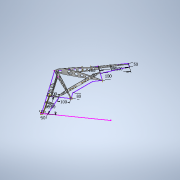
# Autodesk Inventor part: aile1
Saved by Autodesk Inventor 2020 (Build 240168000, 168)
## iProperties
Created: 2019-12-13
Part Number: aile1
Material: Générique
Document SubType Name: Modeling
Designer: guill
Density: 1 g/cm^3
Appearance: Par défaut
Author: guill
Autodesk Inventor part; units mm, degrees
ref_plane "YZ Plane" through (0, 0, 0) normal (1, 0, 0) x (0, 1, 0)
sketch "Esquisse1" plane through (0, 0, 0) normal (0, 1, 0) x (-1, 0, 0)
  line L0 (0, 0) -> (-350.103769, 500)
  line L1 (0, 0) -> (-350.103769, -500)
  line L2 (-350.103769, 500) -> (-178.030838, 254.254387)
  line L3 (-350.103769, -500) -> (-178.030838, -254.254387)
  line L4 (-350.103769, 500) -> (-391.061371, 471.321178)
  line L5 (-350.103769, -500) -> (-391.061371, -471.321178)
  line L6 (-350.103769, 500) -> (-206.70966, 295.211989)
  line L7 (-206.70966, 295.211989) -> (-288.624864, 237.854345)
  line L8 (-288.624864, 237.854345) -> (-391.061371, 471.321178)
  line L9 (-350.103769, -500) -> (-206.70966, -295.211989)
  line L10 (-206.70966, -295.211989) -> (-288.624864, -237.854345)
  line L11 (-288.624864, -237.854345) -> (-391.061371, -471.321178)
  line L12 (-288.624864, 237.854345) -> (-370.540069, 180.496702)
  line L13 (-288.624864, -237.854345) -> (-370.540069, -180.496702)
  line L14 (-370.540069, -180.496702) -> (-324.653954, -114.964538)
  line L15 (-370.540069, 180.496702) -> (-324.653954, 114.964538)
  line L16 (-370.540069, 180.496702) -> (-324.653954, 114.964538)
  line L17 (-324.653954, 114.964538) -> (-324.653954, -114.964538)
  dimension "d19" = 50
  dimension "d20" = 90
  dimension "d21" = 50
  dimension "d22" = 90
  dimension "d23" = 250
  dimension "d24" = 100
  dimension "d25" = 250
  dimension "d26" = 100
  dimension "d27" = 100
  dimension "d28" = 100
  dimension "d29" = 80
  constraints: 36 end point, 4 point on line, 3 perpendicular, 1 vertical
  measures "d19" distance of L0.end L4.end
  measures "d20" angle of L0 L4
  measures "d21" distance of L1.end L5.end
  measures "d22" angle of L1 L5
  measures "d23" distance of L0.end L6.end
  measures "d24" distance of L6.end L7.end
  measures "d25" distance of L1.end L9.end
  measures "d26" distance of L9.end L10.end
  measures "d27" distance of L7.end L12.end
  measures "d28" distance of L10.end L13.end
  measures "d29" distance of L15.end L12.end
ref_plane "Plan de construction11" through (370.540069, 0, 180.496702) normal (0.5735764, 0, 0.819152) x (0.819152, 0, -0.5735764)
sketch "Esquisse3" plane through (370.540069, 0, 180.496702) normal (0.5735764, 0, 0.819152) x (0.819152, 0, -0.5735764)
  line L0 (0, 1) -> (-100, 1)
  line L1 (-200, 0) -> (-200, 1)
  line L2 (-200, 1) -> (-175, 1)
  line L3 (373.576436, 1) -> (-200, 1)
  line L4 (-175, 1) -> (-175, 16)
  line L5 (-175, 16) -> (-193.067438, 16)
  line L6 (-193.067438, 16) -> (-175, 16)
  arc A0 (-175, 16) -> (-200, 1) centre (-175, -12.333333) ccw
  arc A1 (-100, 1) -> (-175, 16) centre (-175, -179) ccw
  line L7 (-175, 1) -> (-175, -4)
  line L8 (-175, -4) -> (-209.42791, -4)
  line L9 (-209.42791, -4) -> (-116.779842, -4)
  arc A2 (-200, 1) -> (-175, -4) centre (-175, 61) ccw
  arc A3 (-175, -4) -> (-100, 1) centre (-175, 561) ccw
  line L10 (-200, 1) -> (-175, 8.5)
  line L11 (-100, 0) -> (-100, 1)
  line L12 (-175, 8.5) -> (-100, 1)
  circle A4 centre (-187, 4.9) radius 5
  circle A5 centre (-163, 7.3) radius 6.5
  circle A6 centre (-148.074442, 5.807444) radius 5.5
  circle A7 centre (-133.074442, 4.307444) radius 4.5
  circle A8 centre (-121.074442, 3.107444) radius 3
  line L13 (-175, 16) -> (-175, 8.5)
  line L14 (-178, 9.840729) -> (-178, 15.840729)
  line L15 (-178, 9.840729) -> (-175, 9.840729)
  line L16 (-175, 16) -> (-175, 9.840729)
  line L17 (-178, 9.840729) -> (-178, -3.895538)
  line L18 (-178, -3.895538) -> (-178, 9.840729)
  line L19 (-175, 9.840729) -> (-175, -4)
  line L20 (-105.241635, 0.322936) -> (-103.229356, 0.322936)
  line L21 (-103.229356, 0.322936) -> (-105.241635, 0.322936)
  line L22 (-105.241635, 0.322936) -> (-105.135598, 0.322936)
  line L23 (-178, 1) -> (-178, -3.895538)
  line L24 (-175, 1) -> (-175, -4)
  line L25 (-178, 1) -> (-178, -3.895538)
  line L26 (-178, -3.603939) -> (-178, 1)
  point P0 (-178, 1)
  point P1 (-175, 9.840729)
  dimension "d36" = 100
  dimension "d37" = 25
  dimension "d38" = 15
  dimension "d40" = 5
  dimension "d94" = 13
  dimension "d95" = 11
  dimension "d96" = 9
  dimension "d97" = 10
  dimension "d98" = 12
  dimension "d99" = 12
  dimension "d100" = 15
  dimension "d101" = 15
  dimension "d102" = 6
  dimension "d103" = 12
  dimension "d104" = 6
  dimension "d105" = 3
  constraints: 48 end point, 14 point on line, 12 point on circle, 9 centre point, 7 collinear, 4 horizontal, 4 tangent, 3 perpendicular, 2 vertical, 1 midpoint, 1 parallel
  measures "d36" distance of L0.start L0.end
  measures "d37" distance of L1.end L2.end
  measures "d38" distance of L2.end L4.end
  measures "d40" distance of L2.end L7.end
  measures "d94" diameter of A5
  measures "d95" diameter of A6
  measures "d96" diameter of A7
  measures "d97" diameter of A4
  measures "d98" distance from line of L4 A4.centre
  measures "d99" distance from line of A5.centre L4
  measures "d100" distance of A5.centre A6.centre
  measures "d101" horizontal distance of A7.centre A6.centre
  measures "d102" diameter of A8
  measures "d103" horizontal distance of A8.centre A7.centre
  measures "d104" distance of L14.start L14.end
  measures "d105" distance of L14.start L15.end
ref_plane "Plan de construction9" through (370.540069, 0, -180.496702) normal (0.5735764, 0, -0.819152) x (-0.819152, 0, -0.5735764)
sketch "Esquisse6" plane through (370.540069, 0, -180.496702) normal (0.5735764, 0, -0.819152) x (-0.819152, 0, -0.5735764)
  point P0 (200, 0)
ref_plane "Plan de construction10" through (0, 1, 0) normal (0, 1, 0) x (1, 0, 0)
sketch "Esquisse7" plane through (0, 1, 0) normal (0, 1, 0) x (1, 0, 0)
  point P0 (0, 0)
ref_plane "Plan de construction12" through (350.103769, 0, 500) normal (0.5735764, 0, 0.819152) x (0.819152, 0, -0.5735764)
sketch "Esquisse9" plane through (350.103769, 0, 500) normal (0.5735764, 0, 0.819152) x (0.819152, 0, -0.5735764)
  line L0 (0.030028, 1) -> (15.030028, 1)
  line L1 (573.576436, 1) -> (0, 1)
  line L2 (0, 0) -> (50, 0)
  line L3 (0, 0) -> (15.030028, 0)
  line L4 (0, 1) -> (50, 1)
  line L5 (15.030028, 0) -> (15.030028, 1)
  dimension "d44" = 15
  constraints: 6 end point, 1 parallel, 1 perpendicular, 1 point on line
  measures "d44" distance of L0.start L0.end
ref_plane "Plan de construction4" through (228.90919, 16, 283.330034) normal (-0.8416187, 0, 0.5400722) x (0, -1, 0)
sketch "Esquisse10" plane through (228.90919, 16, 283.330034) normal (-0.8416187, 0, 0.5400722) x (0, -1, 0)
  ellipse E0 centre (-545, 0) end of major axis (20, 0) minor radius 22.787252 (16, -2.706716) -> (20, 0) ccw
  line L0 (-0.227332, -2.706716) -> (16, -2.706716)
  line L1 (0, -2.997559) -> (0, 0)
  line L2 (0, 0) -> (20, 0)
  line L3 (14.969754, 247.211181) -> (16, 247.211181)
  arc A0 (14.969754, 247.211181) -> (0, 0) centre (1799.771575, 15.074532) ccw
  arc A1 (20, 0) -> (16, 247.211181) centre (-6662.887369, 15.505506) ccw
  line L4 (10, 0) -> (14.969754, 247.211181)
  circle A2 centre (10.265058, 13.184834) radius 6.5
  circle A3 centre (10.667124, 33.184834) radius 6.5
  circle A4 centre (11.049086, 52.184834) radius 6
  circle A5 centre (11.390842, 69.184834) radius 5.5
  circle A6 centre (11.712494, 85.184834) radius 5
  circle A7 centre (12.11456, 105.184834) radius 5
  circle A8 centre (12.436212, 121.184834) radius 4.5
  circle A9 centre (12.737761, 136.184834) radius 4
  circle A10 centre (13.03931, 151.184834) radius 3.5
  circle A11 centre (13.320756, 165.184834) radius 3.5
  circle A12 centre (13.582099, 178.184834) radius 3
  circle A13 centre (14.044474, 201.184834) radius 1.5
  circle A14 centre (13.823338, 190.184834) radius 2.5
  line L5 (1.668204, 94) -> (7.951039, 94)
  line L6 (15, 245.790745) -> (15, -6.022415)
  line L7 (7.951039, 94) -> (7.951039, 97)
  line L8 (7.951039, 97) -> (1.802392, 97)
  ellipse E1 centre (28.333333, 0) end of major axis (0, 0) minor radius 1.142724 (15, 1.008285) -> (0, 0) ccw
  line L9 (15, 1.008285) -> (0, -2.997559)
  line L10 (0, -2.997559) -> (6, -2.997559)
  line L11 (6, -2.997559) -> (6, 0)
  line L12 (0, 0) -> (0, -2.997559)
  ellipse E2 centre (195, 0) end of major axis (0, 0) minor radius 7.864627 (0, 0) -> (15, -3.024856) ccw
  line L13 (0, 0) -> (6, 0)
  line L14 (16, 245.790745) -> (16, -6.022415)
  line L15 (6, 0) -> (6, -2.997559)
  line L16 (15, -3.000658) -> (15, 1.008285)
  line L17 (6, -2.997559) -> (6, 0)
  ellipse E3 centre (28.333333, -2.997559) end of major axis (0, -2.997559) minor radius 1.142724 (15, -1.989274) -> (0, -2.997559) ccw
  line L18 (0, 0) -> (6, 0)
  ellipse E4 centre (195, -2.997559) end of major axis (0, -2.997559) minor radius 7.864627 (0, -2.997559) -> (15, -6.022415) ccw
  line L19 (10, 0) -> (6, 0)
  point P0 (16, -362.083342)
  point P1 (10.134413, 6.686147)
  point P2 (10.395703, 19.683521)
  point P3 (10.536479, 26.686147)
  point P4 (10.797769, 39.683521)
  point P5 (10.928491, 46.186046)
  point P6 (11.169681, 58.183622)
  point P7 (11.280296, 63.685945)
  point P8 (11.501387, 74.683723)
  point P9 (11.611998, 80.185844)
  point P10 (11.81299, 90.183824)
  point P11 (12.014063, 100.185844)
  point P12 (12.215056, 110.183824)
  point P13 (12.345765, 116.685743)
  point P14 (12.526658, 125.683925)
  point P15 (12.657364, 132.185642)
  point P16 (12.818158, 140.184026)
  point P17 (12.968963, 147.685541)
  point P18 (13.109657, 154.684127)
  point P19 (13.250409, 161.685541)
  point P20 (13.391103, 168.684127)
  point P21 (13.521801, 175.18544)
  point P22 (13.642396, 181.184228)
  point P23 (13.77309, 187.685339)
  point P24 (13.873586, 192.684329)
  point P25 (14.014325, 199.685137)
  point P26 (15, 200.02856)
  point P27 (15, 192.390614)
  point P28 (15, 187.979054)
  point P29 (15, 180.828611)
  point P30 (15, 175.541057)
  point P31 (15, 168.255687)
  point P32 (15, 162.113981)
  point P33 (15, 154.084092)
  point P34 (15, 148.285576)
  point P35 (15, 139.483663)
  point P36 (15, 132.886005)
  point P37 (15, 124.883076)
  point P38 (15, 117.486592)
  point P39 (15, 109.268243)
  point P40 (15, 101.101424)
  point P41 (15, 88.952101)
  point P42 (15, 81.417566)
  point P43 (15, 73.335012)
  point P44 (15, 65.034656)
  point P45 (15, 56.700394)
  point P46 (15, 47.669274)
  point P47 (15, 38.030057)
  point P48 (15, 28.339611)
  point P49 (15, 17.63796)
  point P50 (15, 8.731708)
  point P51 (15, 0)
  dimension "d51" = 13
  dimension "d52" = 13
  dimension "d53" = 12
  dimension "d54" = 13.18483
  dimension "d55" = 11
  dimension "d56" = 10
  dimension "d57" = 10
  dimension "d58" = 9
  dimension "d59" = 8
  dimension "d60" = 7
  dimension "d61" = 3
  dimension "d62" = 5
  dimension "d63" = 6
  dimension "d64" = 7
  dimension "d65" = 14
  dimension "d66" = 13
  dimension "d67" = 12
  dimension "d68" = 11
  dimension "d69" = 15
  dimension "d70" = 15
  dimension "d71" = 16
  dimension "d72" = 20
  dimension "d73" = 16
  dimension "d74" = 17
  dimension "d75" = 19
  dimension "d76" = 20
  dimension "d77" = 247.21118
  dimension "d78" = 3
  dimension "d79" = 94
  dimension "d106" = 6
  constraints: 30 end point, 15 centre point, 6 point on circle, 5 horizontal, 4 perpendicular, 3 vertical, 2 collinear, 1 midpoint, 1 parallel, 1 point on line, 22 other
  measures "d51" diameter of A2
  measures "d52" diameter of A3
  measures "d53" diameter of A4
  measures "d54" vertical distance of A2.centre L19.start
  measures "d55" diameter of A5
  measures "d56" diameter of A6
  measures "d57" diameter of A7
  measures "d58" diameter of A8
  measures "d59" diameter of A9
  measures "d60" diameter of A10
  measures "d61" diameter of A13
  measures "d62" diameter of A14
  measures "d63" diameter of A12
  measures "d64" diameter of A11
  measures "d65" vertical distance of A11.centre A10.centre
  measures "d66" vertical distance of A12.centre A11.centre
  measures "d67" vertical distance of A14.centre A12.centre
  measures "d68" vertical distance of A14.centre A13.centre
  measures "d69" vertical distance of A10.centre A9.centre
  measures "d70" vertical distance of A9.centre A8.centre
  measures "d71" vertical distance of A8.centre A7.centre
  measures "d72" vertical distance of A7.centre A6.centre
  measures "d73" vertical distance of A5.centre A6.centre
  measures "d74" vertical distance of A5.centre A4.centre
  measures "d75" vertical distance of A3.centre A4.centre
  measures "d76" vertical distance of A3.centre A2.centre
  measures "d77" distance between parallel lines of L2 L3
  measures "d78" distance from line of L8 L5.start
  measures "d79" distance between parallel lines of L2 L5
  measures "d106" distance of L1.start L10.end
extrude "Extrusion4" add sketch "Esquisse10" along normal blind 3 contours L2 L14 A2 A3 A4 A5 A6 A7 A8 A9 A10 A11 A12 A14 L6 A13 L4 L3 A1 | L2 L6 A2 L14 | L2 L9 L6 | L4 A13 A14 A12 A11 A10 A9 A8 A7 A6 A5 A4 A3 A2 E1 A0 L5 L7 L8 | L11 L10 L9 L0 | L0 L9 E3 L11 | L2 L4 E1 L9 | E1 L4 A2 L6 | A2 L6 A3 L14 | L9 E3 L0 | L0 E3 L9 | E3 L9 E2 L11 | E2 L9 L11 | L2 E1 L4 | L9 E2 L2 L11 | A2 L4 A3 L6 | A13 L6 A14 L4 | E3 L1 L0 | L0 L1 E2 L9 E3 | A3 L6 A4 L14 | A3 L4 A4 L6 | A14 L6 A12 L4 | A4 L6 A5 L14 | A14 L14 A12 L6 | A4 L4 A5 L6 | A12 L6 A11 L4 | A5 L6 A6 L14 | A12 L14 A11 L6 | A5 L4 A6 L6 | A11 L6 A10 L4 | A6 L6 A7 L14 | A11 L14 A10 L6 | A6 L4 A7 L6 | A10 L6 A9 L4 | A7 L6 A8 L14 | A10 L14 A9 L6 | A7 L4 A8 L6 | A9 L6 A8 L4 | A8 L6 A9 L14
sketch "Esquisse11" plane through (279.675976, 8.048961, 362.442192) normal (0.5400722, 0, 0.8416187) x (0.8416187, 0, -0.5400722)
  line L0 (-3, -8.761455) -> (-3, 7.791507)
  line L1 (-3, 6.274364) -> (-3, 6.175837)
  line L2 (66.936248, -8.048961) -> (-22.552672, -8.048961)
  line L3 (-3, 0.174364) -> (-0.027124, 0.174364)
  line L4 (-0.027124, 6.274364) -> (-3, 6.274364)
  line L5 (0, -8.81402) -> (0, 4.18598)
  line L6 (-20.949217, 6.274364) -> (-3, 6.274364)
  line L7 (-39.635584, -7.048961) -> (-15.017799, -7.048961)
  arc A0 (-0.027124, 6.274364) -> (-21.3, -7.048961) centre (-1.513562, -14.996777) ccw
  line L8 (-25.100653, -7.048961) -> (74.817983, -7.048961)
  arc A1 (58.967528, -7.048961) -> (-0.027124, 6.274364) centre (2.642517, -119.178211) ccw
  line L9 (-39.635584, -8.048961) -> (-15.017799, -8.048961)
  line L10 (0, -8.048961) -> (0, -12.066949)
  line L11 (-21.3, -7.048961) -> (-21.3, -8.048961)
  line L12 (-3, -11.509391) -> (0, -11.509391)
  line L13 (6.100773, -11.509391) -> (0, -11.509391)
  arc A2 (-21.3, -8.048961) -> (0, -11.509391) centre (-1.5, 46.541859) ccw
  arc A3 (0, -11.509391) -> (58.967528, -8.048961) centre (2.772798, 445.389574) ccw
  line L14 (58.967528, -7.048961) -> (58.967528, -8.048961)
  ellipse E0 centre (-0.120994, -187.048961) end of major axis (-0.120994, 7.951039) minor radius 194.84134 (74.817983, -7.048961) -> (-0.120994, 7.951039) ccw
  line L15 (0, -1.842696) -> (58.967528, -7.048961)
  circle A4 centre (9, -2.63731) radius 5.5
  circle A5 centre (24, -3.961665) radius 4.5
  circle A6 centre (39, -5.286021) radius 3.5
  line L16 (-21.3, -7.048961) -> (-3, -1.811706)
  line L17 (-3, -8.761455) -> (-3, 1.238545)
  circle A7 centre (-11, -4.101217) radius 4.5
  line L18 (-3, -11.509391) -> (-3, 0.174364)
  line L19 (-0.027124, 0.174364) -> (0, -11.509391)
  line L20 (56.859742, -6.862864) -> (56.859742, -8.048961)
  line L21 (58.967528, -8.048961) -> (56.859742, -8.048961)
  line L22 (56.859742, -6.862864) -> (56.859742, -8.048961)
  point P0 (-24.979659, -7.048961)
  point P1 (-25.100653, -7.048961)
  point P2 (0, -12.048961)
  point P3 (-3, -8.761455)
  point P4 (-3, 0.174364)
  point P5 (-0.008033, -8.048961)
  point P6 (5.545597, -11.509391)
  dimension "d82" = 6.1
  dimension "d83" = 18.3
  dimension "d84" = 11
  dimension "d85" = 9
  dimension "d86" = 7
  dimension "d87" = 15
  dimension "d88" = 15
  dimension "d89" = 9
  dimension "d90" = 8
  dimension "d91" = 9
  constraints: 30 end point, 14 point on line, 11 point on circle, 8 centre point, 5 perpendicular, 4 vertical, 2 collinear, 1 horizontal, 6 other
  measures "d82" distance of L1.start L3.start
  measures "d83" distance between parallel lines of L0 L11
  measures "d84" diameter of A4
  measures "d85" diameter of A5
  measures "d86" diameter of A6
  measures "d87" horizontal distance of A5.centre A4.centre
  measures "d88" horizontal distance of A6.centre A5.centre
  measures "d89" diameter of A7
  measures "d90" distance from line of A7.centre L17
extrude "Extrusion5" add sketch "Esquisse11" along normal blind 3 contours L16 A7 A0 L0 | L0 L8 A7 L16 | L0 L4 A1 L15 A6 A5 A4 L5 L8 L19 L3 | L0 L2 A7 L8 | L0 L18 A2 L2 A7 | L8 L5 L2 L19 | A7 L8 L7 L16 | A7 L2 L11 L7 L8 | L8 A4 L2 L5 | L5 L15 A4 L8 | L2 A4 A5 A6 A3 L13 L10 L5 | A4 L15 A5 L8 | L8 A5 L2 A4 | L20 L2 A6 L8 | L8 A6 L15 L20 | A5 L15 A6 L8 | L8 A6 L2 A5
extrude "Extrusion6" add sketch "Esquisse3" along normal blind 3 contours L17 L10 L4 L2 | L2 L7 A2 A4 | L2 A4 L10 L17 | L4 L12 A5 L3 | L3 A5 A6 A7 A8 A3 L7 | L17 L15 L4 L10 | L10 A4 A0 L14 L17 | L4 A1 L12 A8 A7 A6 A5 | L2 L10 A4 | A5 L12 A6 L3 | L3 A8 L12 | A6 L12 A7 L3 | L3 A7 L12 A8 picked at (-194.398279, 2.332998) picked at (-112.107283, 1.985135)
ref_plane "Plan de construction5" through (0, 1, 0) normal (0.4379247, 0, -0.8990117) x (0.8990117, 0, 0.4379247)
sketch "Esquisse12" plane through (0, 1, 0) normal (0.4379247, 0, -0.8990117) x (0.8990117, 0, 0.4379247)
  line L0 (0, 0) -> (315.115011, 0)
  line L1 (0, 0) -> (90, 0)
  line L2 (90, 0) -> (90, -40)
  line L3 (0, 1) -> (0, 0)
  line L4 (0, 0) -> (90, 0)
  line L5 (90, 1) -> (90, 16)
  line L6 (90, -40) -> (64.056463, -40)
  arc A0 (0, 0) -> (90, -40) centre (90, 81.25) ccw
  line L7 (90, 16) -> (68.484817, 16)
  arc A1 (90, 16) -> (0, 1) centre (86.556789, -240.840731) ccw
  line L8 (90, -40) -> (109.634057, -40)
  line L9 (363.639408, 1) -> (412.163805, 1)
  arc A2 (90, -40) -> (412.163805, 1) centre (99.817028, 1169.087008) ccw
  line L10 (90, 16) -> (104.02297, 16)
  line L11 (0, 0) -> (90, -17.116159)
  line L12 (90, -17.116159) -> (384.32761, 1)
  line L13 (412.163805, 1) -> (342.2135, 1)
  circle A3 centre (50, -9.508977) radius 16.5
  circle A4 centre (135, -14.346364) radius 20
  circle A5 centre (190, -10.961059) radius 15
  circle A6 centre (237.163805, -8.05808) radius 13.5
  circle A7 centre (282.163805, -5.288285) radius 12.5
  circle A8 centre (322.163805, -2.826244) radius 8.5
  line L14 (412.163805, 1) -> (412.163805, 0)
  line L15 (90, 0) -> (90, 21.872289)
  line L16 (0, 1) -> (399.114343, 1)
  line L17 (90, 16) -> (105.35625, 16)
  line L18 (105.35625, 16) -> (90, 16)
  arc A9 (412.163805, 1) -> (90, 16) centre (97.011485, -3300.56079) ccw
  line L19 (314.469379, -20.834055) -> (314.469379, -10.834055)
  line L20 (314.469379, -10.834055) -> (311.469379, -10.834055)
  line L21 (311.469379, -10.834055) -> (311.469379, -21.371328)
  point P0 (104.02297, 16)
  point P1 (83.113577, 16)
  dimension "d110" = 90
  dimension "d111" = 315.11501
  dimension "d112" = 40
  dimension "d113" = 90
  dimension "d114" = 90
  dimension "d115" = 15
  dimension "d116" = 33
  dimension "d117" = 40
  dimension "d118" = 45
  dimension "d119" = 30
  dimension "d120" = 55
  dimension "d121" = 40
  dimension "d122" = 27
  dimension "d123" = 25
  dimension "d124" = 17
  dimension "d126" = 40
  dimension "d127" = 45
  dimension "d128" = 90
  dimension "d167" = 10
  dimension "d169" = 3
  constraints: 32 end point, 12 point on circle, 10 centre point, 9 point on line, 4 horizontal, 4 vertical, 3 collinear, 2 perpendicular, 1 midpoint, 1 tangent, 1 other
  measures "d110" distance of L0.start L1.end
  measures "d111" distance of L0.start L0.end
  measures "d112" distance of L1.end L2.end
  measures "d113" distance from line of L5 L3.start
  measures "d114" angle of L0 L5
  measures "d115" distance of L5.start L5.end
  measures "d116" diameter of A3
  measures "d117" distance from line of L2 A3.centre
  measures "d118" distance from line of A4.centre L2
  measures "d119" diameter of A5
  measures "d120" horizontal distance of A4.centre A5.centre
  measures "d121" diameter of A4
  measures "d122" diameter of A6
  measures "d123" diameter of A7
  measures "d124" diameter of A8
  measures "d126" horizontal distance of A8.centre A7.centre
  measures "d127" horizontal distance of A7.centre A6.centre
  measures "d167" distance of L19.start L19.end
  measures "d169" distance of L19.end L20.end
extrude "Extrusion7" add sketch "Esquisse12" along normal blind 3 contours L3 L16 A3 L0 | L11 A3 L2 A0 | L0 A3 L11 | A1 L7 L5 L16 A3 | L2 L12 A4 A5 A6 A7 A8 L9 A2 L19 L20 L21 L8 | A3 L16 L15 L0 | L0 L2 L11 A3 | L2 L0 A4 L12 | L15 L16 A4 L0 | L10 A9 L9 L13 L16 A8 A7 A6 A5 A4 L5 | A4 L0 A5 L12 | A4 L16 A5 L0 | A5 L0 A6 L12 | A5 L16 A6 L0 | L12 A8 L16 L13 L9 | A6 L0 A7 L12 | A6 L16 A7 L0 | L12 A7 L0 A8 | L0 A7 L16 A8 picked at (22.726983, -3.529396)
sketch3d "Esquisse 3D4"
ref_plane "Plan de construction6" through (130.905839, 0, 186.952914) normal (-0.819152, 0, 0.5735764) x (0.5735764, 0, 0.819152)
ref_plane "Plan de construction7" through (163.671921, 0, 164.009856) normal (-0.819152, 0, 0.5735764) x (0.5735764, 0, 0.819152)
sketch "Esquisse14" plane through (163.671921, 0, 164.009856) normal (-0.819152, 0, 0.5735764) x (0.5735764, 0, 0.819152)
  ellipse E0 centre (-150.989006, -80.25) end of major axis (-150.989006, 41) minor radius 106.01843 (-150.989006, 41) -> (-229.683098, 1) ccw
  line L0 (-92.698652, 1) -> (-170.081176, 1)
  line L1 (132.159928, -4) -> (132.159928, 0)
  line L2 (-155.554616, -15) -> (-157.010348, -15)
  arc A0 (-155.554616, -15) -> (132.159928, -4) centre (-365.037985, 9232.431054) ccw
  line L3 (135.159928, -4) -> (135.159928, 0)
  line L4 (-155.76889, 15.116385) -> (132.159928, 6)
  circle A1 centre (-118.073259, 13.922868) radius 20
  circle A2 centre (-68.073259, 12.339771) radius 17.5
  circle A3 centre (-23.073259, 10.914984) radius 17.5
  circle A4 centre (16.926741, 9.648506) radius 15
  circle A5 centre (51.926741, 8.540338) radius 12.5
  circle A6 centre (86.926741, 7.43217) radius 10
  line L5 (-155.952102, 40.867067) -> (-155.554616, -15)
  line L6 (132.164808, 16) -> (132.043814, 16)
  line L7 (135.159928, 6.107444) -> (132.159928, 6.107444)
  line L8 (132.159928, -4) -> (135.159928, -4)
  line L9 (132.159928, -4) -> (132.159928, 6)
  line L10 (135.159928, 13.8) -> (132.159928, 13.8)
  line L11 (132.159928, 6.107444) -> (132.164808, 16)
  line L12 (132.159928, 1) -> (132.159928, 16)
  arc A7 (132.159928, 16) -> (-155.952102, 40.867067) centre (-142.376027, -1483.31855) ccw
  point P0 (-228.227366, 0)
  point P1 (-92.698652, 15.346364)
  point P2 (-170.081176, 10.508977)
  dimension "d132" = 40
  dimension "d135" = 35
  dimension "d136" = 35
  dimension "d137" = 30
  dimension "d138" = 25
  dimension "d139" = 20
  dimension "d140" = 50
  dimension "d141" = 45
  dimension "d142" = 40
  dimension "d143" = 35
  dimension "d144" = 35
  constraints: 11 end point, 8 centre point, 7 point on line, 4 point on circle, 2 other
  measures "d132" diameter of A1
  measures "d135" diameter of A2
  measures "d136" diameter of A3
  measures "d137" diameter of A4
  measures "d138" diameter of A5
  measures "d139" diameter of A6
  measures "d140" horizontal distance of A1.centre A2.centre
  measures "d141" horizontal distance of A2.centre A3.centre
  measures "d142" horizontal distance of A3.centre A4.centre
  measures "d143" horizontal distance of A5.centre A4.centre
  measures "d144" horizontal distance of A5.centre A6.centre
extrude "Extrusion8" add sketch "Esquisse14" along normal blind 3 contours A1 L4 A2 A3 A4 A5 A6 L9 L1 A0 L5 L0 | L0 L5 L4 A1 | A1 L4 L5 A7 L12 A6 A5 A4 A3 A2
ref_plane "Plan de construction8" through (279.653954, 0, 114.964538) normal (1, 0, 0) x (0, 0, -1)
sketch "Esquisse17" plane through (279.653954, 0, 114.964538) normal (1, 0, 0) x (0, 0, -1)
  line L0 (-20.233507, 21.861581) -> (251.179948, 21.861581)
  line L1 (251.179948, 21.861581) -> (251.179948, 11.861581)
  line L2 (251.179948, 11.861581) -> (248.179948, 11.861581)
  line L3 (248.179948, 11.861581) -> (248.179948, -8.138419)
  line L4 (-20.233507, 21.861581) -> (6.05195, 21.861581)
  line L5 (-20.233507, 21.861581) -> (-20.233507, 11.861581)
  line L6 (-20.233507, 11.861581) -> (-17.233507, 11.861581)
  line L7 (-17.233507, 11.861581) -> (-17.233507, -8.138419)
  line L8 (-17.233507, -8.138419) -> (248.179948, -8.138419)
  line L9 (-17.233507, 5.661217) -> (248.179948, 5.436761)
  circle A0 centre (14.766493, 5.634155) radius 11
  circle A1 centre (44.766493, 5.617997) radius 11
  circle A2 centre (74.766493, 5.583414) radius 11
  circle A3 centre (156.179948, 5.514564) radius 11
  circle A4 centre (186.179948, 5.489194) radius 11
  circle A5 centre (216.179948, 5.463823) radius 11
  point P0 (114.964538, 0)
  dimension "d148" = 10
  dimension "d149" = 20
  dimension "d150" = 3
  dimension "d151" = 10
  dimension "d152" = 3
  dimension "d153" = 32
  dimension "d154" = 22
  dimension "d155" = 22
  dimension "d156" = 22
  dimension "d157" = 22
  dimension "d158" = 22
  dimension "d159" = 22
  dimension "d160" = 32
  dimension "d161" = 30
  dimension "d162" = 30
  dimension "d163" = 30
  dimension "d164" = 30
  constraints: 20 end point, 7 point on line, 6 centre point, 4 perpendicular, 1 collinear, 1 parallel, 1 vertical
  measures "d148" distance of L0.end L1.end
  measures "d149" distance of L2.end L3.end
  measures "d150" distance of L1.end L2.end
  measures "d151" distance of L0.start L5.end
  measures "d152" distance of L5.end L6.end
  measures "d153" distance from line of L3 A5.centre
  measures "d154" diameter of A5
  measures "d155" diameter of A4
  measures "d156" diameter of A3
  measures "d157" diameter of A2
  measures "d158" diameter of A1
  measures "d159" diameter of A0
  measures "d160" distance from line of A0.centre L7
  measures "d161" distance of A0.centre A1.centre
  measures "d162" distance of A2.centre A1.centre
  measures "d163" distance of A5.centre A4.centre
  measures "d164" distance of A4.centre A3.centre
extrude "Extrusion9" add sketch "Esquisse17" along normal blind 3 contours L0 L1 L2 L3 L9 A5 A4 A3 A2 A1 A0 L7 L6 L5 | L9 A0 A1 A2 A3 A4 A5 L3 L8 L7
sketch "Esquisse18" plane through (279.653954, 0, 114.964538) normal (-1, 0, 0) x (0, 0, 1)
  ellipse E0 centre (-395.837116, -179) end of major axis (-395.837116, 16) minor radius 111.847405 (-352.818883, 1) -> (-387.23347, 15.422221) ccw
  arc A0 (-250.314404, 21.779022) -> (-359.107055, 5.185435) centre (-217.439426, -558.695234) ccw
  line L0 (-359.107055, 5.185435) -> (-359.107055, 0.774363)
  line L1 (-250.314404, 21.779022) -> (-250.314404, -8.220978)
  ellipse E1 centre (-157.448261, 3301.56079) end of major axis (-157.448261, -15.007411) minor radius 1452.407063 (-295.46124, 0) -> (-160.518764, -15) ccw
  arc A1 (-359.107055, 0.774363) -> (-250.314404, -8.220978) centre (-261.121757, 523.456267) ccw
  line L2 (-359.107055, 2.979899) -> (-250.314404, 6.779022)
  circle A2 centre (-270.314404, 6.080607) radius 11
  circle A3 centre (-295.467248, 5.20225) radius 0
  circle A4 centre (-309.107055, 4.725938) radius 8.5
  line L3 (-296.107055, 14.245123) -> (-286.107055, 14.245123)
  line L4 (-286.107055, 14.245123) -> (-286.107055, -4.991942)
  line L5 (-286.107055, -4.991942) -> (-296.107055, -4.991942)
  line L6 (-296.107055, -4.991942) -> (-296.107055, 14.245123)
  point P0 (-114.964538, 0)
  dimension "d170" = 30
  dimension "d171" = 17
  dimension "d172" = 22
  dimension "d173" = 20
  dimension "d174" = 50
  dimension "d175" = 10
  dimension "d176" = 2
  dimension "d177" = 13
  constraints: 14 end point, 5 centre point, 4 point on circle, 3 parallel, 3 point on line, 2 midpoint, 1 horizontal, 1 perpendicular, 1 tangent, 1 vertical, 4 other
  measures "d170" distance of L1.start L1.end
  measures "d171" diameter of A4
  measures "d172" diameter of A2
  measures "d173" distance from line of L1 A2.centre
  measures "d174" distance from line of L0 A4.centre
  measures "d175" distance between parallel lines of L4 L6
  measures "d176" angle of L2 L5
  measures "d177" distance from line of A4.centre L6
sketch "Esquisse18 outline for Extrusion10" plane through (279.653954, 0, 114.964538) normal (-1, 0, 0) x (0, 0, 1)
  line L0 (-250.314404, -8.220978) -> (-250.314404, 21.779022)
  arc A0 (-359.107055, 0.774363) -> (-250.314404, -8.220978) centre (-261.121757, 523.456267) ccw
  arc A1 (-250.314404, 21.779022) -> (-359.107055, 5.185435) centre (-217.439426, -558.695234) ccw
  line L1 (-359.107055, 5.185435) -> (-359.107055, 0.774363)
  circle A2 centre (-309.107055, 4.725938) radius 8.5
  line L2 (-286.107055, 14.245123) -> (-286.107055, -4.991942)
  line L3 (-296.107055, 14.245123) -> (-286.107055, 14.245123)
  line L4 (-296.107055, -4.991942) -> (-296.107055, 14.245123)
  line L5 (-286.107055, -4.991942) -> (-296.107055, -4.991942)
  circle A3 centre (-270.314404, 6.080607) radius 11
extrude "Extrusion10" add sketch "Esquisse18 outline for Extrusion10" against normal blind 3
ref_plane "Plan de construction13" through (202.603699, 7.3, -224.840538) normal (-0.5735764, 0, 0.819152) x (0.819152, 0, 0.5735764)
sketch "Esquisse19" plane through (202.603699, 7.3, -224.840538) normal (-0.5735764, 0, 0.819152) x (0.819152, 0, 0.5735764)
  line L0 (0.078389, 18.672773) -> (-4.971803, 18.672773)
  line L1 (0, -14.327227) -> (-5.234817, -14.327227)
  arc A0 (0.078389, 18.672773) -> (-37, -7.3) centre (0.078389, -20.779924) ccw
  arc A1 (-37, -7.3) -> (0, -14.327227) centre (-1.754499, 77.355376) ccw
  line L2 (0.078389, 18.672773) -> (3, 18.672773)
  line L3 (3, 8.672773) -> (0, 8.672773)
  line L4 (0, 8.672773) -> (0, -14.327227)
  line L5 (3, 18.672773) -> (3, 8.672773)
  line L6 (-37, -7.3) -> (0, 5.607636)
  line L7 (0, 10.13217) -> (0, -9.86783)
  circle A2 centre (-15, 0.374811) radius 9
  point P0 (0, 33.567067)
  point P1 (3, 33.567067)
  point P2 (-3.508999, -14.327227)
  dimension "d181" = 10
  dimension "d182" = 18
  dimension "d183" = 15
  dimension "d184" = 3
  dimension "d185" = 23
  constraints: 14 end point, 5 point on circle, 3 centre point, 3 horizontal, 2 point on line, 1 parallel, 1 perpendicular, 1 tangent, 1 vertical
  measures "d181" distance of L2.end L3.start
  measures "d182" diameter of A2
  measures "d183" distance from line of L4 A2.centre
  measures "d184" distance of L3.start L3.end
  measures "d185" distance of L3.end L1.start
extrude "Extrusion11" add sketch "Esquisse19" along normal blind 3 contours L1 A1 L6 A2 L4 | A0 L2 L5 L3 L4 L6 A2
ref_plane "Plan de construction14" through (161.306196, 7.3, -165.861591) normal (-0.5735764, 0, 0.819152) x (0.819152, 0, 0.5735764)
sketch "Esquisse20" plane through (161.306196, 7.3, -165.861591) normal (-0.5735764, 0, 0.819152) x (0.819152, 0, 0.5735764)
  arc A0 (-0.368419, 26.759232) -> (-37, -7.3) centre (5.238237, -15.99959) ccw
  line L0 (-0.368419, 26.759232) -> (2.631581, 26.759232)
  line L1 (2.631581, 16.759232) -> (2.631581, 26.759232)
  line L2 (2.631581, 16.759232) -> (-0.368419, 16.759232)
  line L3 (-0.368419, 16.759232) -> (-0.368419, -17.898506)
  arc A1 (-37, -7.3) -> (-0.368419, -17.898506) centre (-0.786573, 49.260288) ccw
  line L4 (-37, -7.3) -> (-0.368419, 7.806724)
  circle A2 centre (-15.368419, 1.620781) radius 11.5
  point P0 (0, 33.567067)
  point P1 (3, 33.567067)
  dimension "d189" = 3
  dimension "d190" = 10
  dimension "d191" = 34.65774
  dimension "d192" = 23
  dimension "d193" = 15
  constraints: 10 end point, 4 point on circle, 3 centre point, 2 horizontal, 2 point on line, 1 parallel, 1 perpendicular
  measures "d189" distance of L1.start L2.end
  measures "d190" distance of L1.start L0.end
  measures "d191" distance of L2.end L3.end
  measures "d192" diameter of A2
  measures "d193" distance from line of L3 A2.centre
extrude "Extrusion12" add sketch "Esquisse20" along normal blind 3 contours L0 L1 L2 L3 L4 A2 A0 | L4 A2 L3 A1
mirror "Symétrie4" about plane through (0, 0, 0) normal (0, 0, 1)
